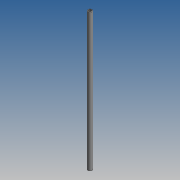
# Autodesk Inventor part: P046_AxeCouvercleFretté
Saved by Autodesk Inventor 2021.3 (Build 253353000, 353)
## iProperties
Created: 2022-01-08
Part Number: P046_AxeCouvercleFretté
Material: Générique
Document SubType Name: Modeling
Designer: gabri
Density: 1 g/cm^3
Appearance: Par défaut
Author: gabri
Autodesk Inventor part; units mm, degrees
ref_plane "YZ Plane" through (0, 0, 0) normal (1, 0, 0) x (0, 1, 0)
ref_plane "XZ Plane" through (0, 0, 0) normal (0, 1, 0) x (-1, 0, 0)
ref_plane "XY Plane" through (0, 0, 0) normal (0, 0, 1) x (1, 0, 0)
sketch "Sketch3" plane through (0, 0, 0) normal (0, 0, 1) x (1, 0, 0)
  circle A0 centre (0, 0) radius 3
  circle A1 centre (0, 0) radius 2
  dimension "d10" = 4
  dimension "d11" = 6
  constraints: 2 centre point, 2 coincident
  measures "d10" diameter of A1
  measures "d11" diameter of A0
extrude "Extrusion1" add sketch "Sketch3" along normal blind 200
thread "Thread2" size "M4x0.7" class "6H" standard "ISO Metric profile" length 10
thread "Thread3" size "M4x0.7" class "6H" standard "ISO Metric profile" length 10
fillet "Fillet1" radius 0.5 2 edges at (-3, 0, 0) (-3, 0, 200)
body "Solid2"
